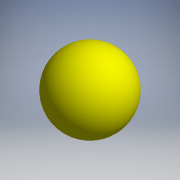
# Autodesk Inventor part: SKF_W 61701-2RS1_PART3
Saved by Autodesk Inventor 2021.3 (Build 253353000, 353)
## iProperties
Part Number: SKF_W 61701-2RS1_PART3
Material: Generic
Catalog Web Link: www.cadenas.de
Description: -Deep groove ball bearings
Vendor: SKF
Document SubType Name: Modeling
Designer: partserver
Manufacturer: SKF
Mass: 3 g
Surface Area: 0.0792229 cm^2
Volume: 0.00209677 cm^3
Density: 1 g/cm^3
Appearance: PSOLRGB-192-192-192
Category: PARTsolutions
Company: SKF
PSOL_IDENT_0: {$CADENAS_DATA\23d-libs\skf\bearings_units_and_housings\ball_bearings\deep_groove_ball_bearings\bb1_
PSOL_IDENT_1: 001_101.prj},211 {VTYP=3D},{NB=SKF_W 61701-2RS1_PART3},{LINA=SKF_W 61701-2RS1_PART3},{NN=BB1_001_101
PSOL_IDENT_2: _PART3},{NOPRJ=TRUE},{DATE=13.05.2022 09:20:28},{GEOMDATE=02.05.2022 07:22:49},{VERSION=},{LINEID=16
PSOL_IDENT_3: 210},{WBVAR=},{WBNUMERIC=}  {NB=SKF_W 61701-2RS1_PART3},{LINA=SKF_W 61701-2RS1_PART3},{KT=DUMMY},{DE
PSOL_IDENT_4: SIGNATION=W 61701-2RS1},{R12=0.20},{DD=12.000},{D=18.000},{B=4.000},{C=},{CX=},{CXX=},{CA=0.000},{XX
PSOL_IDENT_5: VARIANT=},{XXDESIGN=Single row stainless steel},{XXSEALING=Contact seal on both sides},{DESIGN=dgbbw
PSOL_IDENT_6: 2rs},{DESIGNIR=dgbbw2rs},{VARIANT=},{DD1=13.86},{DD2=13.86},{DD2X=},{DD2A=13.86},{D1=16.10},{D1X=0.0
PSOL_IDENT_7: 0},{D2=16.7},{D2A=16.70},{D3=},{D3X=},{D3A=0.000},{D4=},{HH=0.000},{BB=0.000},{BBX=},{BBA=0.000},{FF=
PSOL_IDENT_8: },{R0MAX=0.000},{R0=0.000},{PITCH=15.00},{DW=1.588},{DDAMIN=13.500},{DDAMAX=13.500},{DDBMIN=0.000},{
PSOL_IDENT_9: DDBMAX=0.000},{DBMIN=0.000},{DAMAX=17.000},{BBAMIN=0.000},{CAMAX=0.000},{RAMAX=0.200},{LOAD1=0.527},
PSOL_IDENT_10: {LOAD2=0.265},{LOAD3=0.011},{SPEED1=0},{SPEED2=22000},{KR=0.015},{F0=8.200},{Z=13},{II=1},{MASS=0.00
PSOL_IDENT_11: 3},{BEARING=W 61701-2RS1},{RING=},{HELP=0.950},{HELP2=0.650},{DD1ALG=6.930},{YALG=6.930},{PITCH1=15.
PSOL_IDENT_12: 000},{DW1=1.588},{YALG1=8.050},{HALG1=0.950},{SH=6.930},{CU=0.482},{HALG=0.93},{B1=0},{SHIELDHELP=2}
PSOL_IDENT_13: ,{D4A=0.000},{FFA=0.000},{RS1=},{HELP3=0}
NB: SKF_W 61701-2RS1_PART3
NT: Deep groove ball bearings
NBSYN: SKF_$DESIGNATION._PART3
LINA: SKF_W 61701-2RS1_PART3
CATALOG: SKF
DESIGNATION: W 61701-2RS1
R12: 0.2
DD: 12
D: 18
B: 4
XXDESIGN: Single row stainless steel
XXSEALING: Contact seal on both sides
DD2: 13.86
D2: 16.7
LOAD1: 0.527
LOAD2: 0.265
LOAD3: 0.011
SPEED1: 0
SPEED2: 22000
BEARING: W 61701-2RS1
SUPPLIER: SKF
ARTICLENO: SKF_W 61701-2RS1_PART3
BOMINFO: SKF_W 61701-2RS1_PART3
CREATOR: CADENAS GmbH
Title: SKF_W 61701-2RS1_PART3
Author: Cadenas PARTsolutions
Comments: Deep groove ball bearings
Autodesk Inventor part; units mm, degrees
ref_plane "YZ Plane" through (0, 0, 0) normal (1, 0, 0) x (0, 1, 0)
ref_plane "XZ Plane" through (0, 0, 0) normal (0, 1, 0) x (-1, 0, 0)
ref_plane "XY Plane" through (0, 0, 0) normal (0, 0, 1) x (1, 0, 0)
sketch "Sketch_6" plane through (0, 0, 0) normal (0, 0, 1) x (1, 0, 0)
  line L0 (2.794, 7.5) -> (1.206, 7.5)
  arc A0 (2.794, 7.5) -> (1.206, 7.5) centre (2, 7.5) ccw
  line L1 (2.794, 7.5) -> (1.206, 7.5)
  dimension "d0" = 360
  constraints: 4 end point, 2 point on circle, 1 centre point
revolve "Revolution1" add sketch "Sketch_6" angle 360 about axis through (2.794, 7.5, 0) along (1, 0, 0)
body "Solid1"
